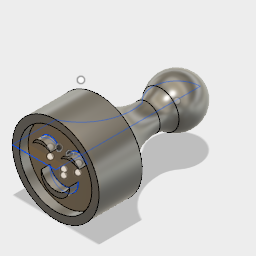
yinzhang (Autodesk Fusion 360 design; units mm, degrees)
Autodesk Fusion 360 part; units mm, degrees
note: some values were not read from the file. Set by a fixed rule: which sketch regions a step uses.
sketch "草图1" plane through (0, 0, 0) normal (0, 1, 0) x (1, 0, 0)
  arc A0 (10, 0) -> (5, -15) centre (10.368, -8.456) ccw
  arc A1 (-5, -35) -> (5, -15) centre (-12.5094, -18.7453) ccw
  line L0 (-5, -35) -> (-5, -50)
  line L1 (-5, -50) -> (10, -50)
  line L2 (10, -50) -> (10, 0)
revolve "旋转1" add sketch "草图1" angle 360 about axis through (10, 0, 50) along (0, 0, -1)
fillet "圆角1" radius 8 1 edges at (5.3384, 1.8081, 15)
sketch "草图2" plane through (0, 0, 50) normal (0, 0, 1) x (1, 0, 0)
  circle A0 centre (10, 0) radius 15
  circle A1 centre (10, 0) radius 12.5
  dimension "d3" = 25
  measures "d3" diameter of A1
extrude "拉伸1" cut sketch "草图2" against normal blind 3 contours A1
sketch "草图3" plane through (0, 0, 47) normal (0, 0, 1) x (1, 0, 0)
  circle A0 centre (10, 0) radius 12.5
  arc A1 (8.1538, 4.2198) -> (2, 4) centre (5.1209, 2.8791) ccw
  arc A2 (8.1538, 4.2198) -> (2, 4) centre (5.2193, 0.1235) ccw
  arc A3 (18, 4) -> (11.8616, 4.2131) centre (14.8887, 2.8928) ccw
  arc A4 (18, 4) -> (11.8616, 4.2131) centre (14.7934, 0.1488) ccw
  arc A5 (5.0394, -2.3356) -> (14.7934, -2.7249) centre (9.9673, -1.2563) ccw
  arc A6 (5.0394, -2.3356) -> (14.7934, -2.7249) centre (9.8914, -3.1578) ccw
extrude "拉伸2" add sketch "草图3" along normal blind 3 contours A5 A6
extrude "拉伸3" add sketch "草图3" along normal blind 3 contours A1 A2
extrude "拉伸4" add sketch "草图3" along normal blind 3 contours A3 A4
